Autodesk Fusion 360 part; units mm, degrees
note: some values were not read from the file. Set by a fixed rule: which sketch regions a step uses.
(part 13 of 15)
  line L10593 (41.7362, -55.8779) -> (41.8637, -56.1141)
  line L10594 (295.811, -57.5311) -> (295.669, -57.7588)
  line L10595 (295.496, -57.9642) -> (295.297, -58.1433)
  line L10596 (38.2329, -56.8363) -> (38.2603, -56.5693)
  line L10597 (42.0283, -57.0153) -> (41.9925, -57.2813)
  line L10598 (120.911, -58.0691) -> (121.001, -57.9066)
  line L10599 (41.3885, -55.4708) -> (41.5768, -55.662)
  line L10600 (292.292, -57.1145) -> (292.243, -56.8505)
  line L10601 (293.517, -58.4396) -> (293.269, -58.3349)
  line L10602 (-14.6725, -54.4815) -> (-14.3973, -54.5453)
  line L10603 (293.139, -55.022) -> (293.377, -54.8983)
  line L10604 (292.233, -56.5823) -> (292.26, -56.3153)
  line L10605 (-13.8873, -54.7853) -> (-13.6627, -54.9567)
  line L10606 (292.561, -55.574) -> (292.727, -55.3633)
  line L10607 (292.921, -55.178) -> (293.139, -55.022)
  line L10608 (292.377, -57.3691) -> (292.292, -57.1145)
  line L10609 (293.269, -58.3349) -> (293.039, -58.1965)
  line L10610 (295.297, -58.1433) -> (295.073, -58.2924)
  line L10611 (294.042, -58.5399) -> (293.776, -58.5083)
  line L10612 (294.311, -58.5336) -> (294.042, -58.5399)
  line L10613 (-14.3973, -54.5453) -> (-14.1338, -54.6473)
  line L10614 (292.727, -55.3633) -> (292.921, -55.178)
  line L10615 (292.497, -57.6092) -> (292.377, -57.3691)
  line L10616 (293.631, -54.8093) -> (293.894, -54.757)
  line L10617 (294.162, -54.7422) -> (294.429, -54.7654)
  line L10618 (-13.1625, -55.6339) -> (-13.0648, -55.8989)
  line L10619 (-13.0648, -55.8989) -> (-13.0053, -56.1751)
  line L10620 (-13.9944, -58.1942) -> (-14.2491, -58.3165)
  line L10621 (-16.5462, -57.7074) -> (-16.7068, -57.475)
  line L10622 (-16.7068, -57.475) -> (-16.8331, -57.2223)
  line L10623 (292.325, -56.0549) -> (292.426, -55.8061)
  line L10624 (292.26, -56.3153) -> (292.325, -56.0549)
  line L10625 (293.894, -54.757) -> (294.162, -54.7422)
  line L10626 (-13.1036, -57.1344) -> (-13.2178, -57.3928)
  line L10627 (-16.9225, -56.9543) -> (-16.9733, -56.6764)
  line L10628 (-13.5491, -57.8487) -> (-13.7595, -58.0372)
  line L10629 (293.776, -58.5083) -> (293.517, -58.4396)
  line L10630 (-14.2491, -58.3165) -> (-14.5185, -58.4016)
  line L10631 (294.576, -58.4895) -> (294.311, -58.5336)
  line L10632 (-16.8331, -57.2223) -> (-16.9225, -56.9543)
  line L10633 (-16.9733, -56.6764) -> (-16.9844, -56.3941)
  line L10634 (-16.9844, -56.3941) -> (-16.9556, -56.1131)
  line L10635 (-16.9556, -56.1131) -> (-16.8875, -55.8389)
  line L10636 (293.377, -54.8983) -> (293.631, -54.8093)
  line L10637 (39.6306, -55.0633) -> (39.8939, -55.011)
  line L10638 (295.577, -55.408) -> (295.736, -55.6239)
  line L10639 (293.039, -58.1965) -> (292.831, -58.027)
  line L10640 (295.073, -58.2924) -> (294.831, -58.4086)
  line L10641 (-13.0053, -56.1751) -> (-12.9853, -56.4569)
  line L10642 (292.831, -58.027) -> (292.649, -57.83)
  line L10643 (294.831, -58.4086) -> (294.576, -58.4895)
  line L10644 (-13.4645, -55.158) -> (-13.2967, -55.3853)
  line L10645 (-14.1338, -54.6473) -> (-13.8873, -54.7853)
  line L10646 (-16.8875, -55.8389) -> (-16.7814, -55.577)
  line L10647 (295.175, -55.054) -> (295.388, -55.2168)
  line L10648 (292.243, -56.8505) -> (292.233, -56.5823)
  line L10649 (292.649, -57.83) -> (292.497, -57.6092)
  line L10650 (292.426, -55.8061) -> (292.561, -55.574)
  line L10651 (38.2435, -57.1045) -> (38.2329, -56.8363)
  line L10652 (-9.0561, -57.5495) -> (-9.1147, -57.7254)
  line L10653 (-15.7796, -54.6214) -> (-15.5131, -54.5278)
  line L10654 (-9.0329, -57.3656) -> (-9.0561, -57.5495)
  line L10655 (-15.8933, -58.2389) -> (-16.1354, -58.0932)
  line L10656 (-13.7595, -58.0372) -> (-13.9944, -58.1942)
  line L10657 (-13.6627, -54.9567) -> (-13.4645, -55.158)
  line L10658 (-13.3673, -57.6325) -> (-13.5491, -57.8487)
  line L10659 (-10.5247, -58.1191) -> (-10.6659, -57.999)
  line L10660 (-16.6395, -55.3327) -> (-16.4646, -55.1109)
  line L10661 (-9.4735, -58.1412) -> (-9.639, -58.2248)
  line L10662 (-10.7811, -57.8537) -> (-10.8658, -57.6888)
  line L10663 (-9.1913, -56.8133) -> (-9.1042, -56.977)
  line L10664 (160.061, -56.6385) -> (160.163, -56.7784)
  line L10665 (-9.9759, -56.3891) -> (-9.7915, -56.4084)
  line L10666 (-9.0506, -57.1545) -> (-9.0325, -57.339)
  line L10667 (160.25, -57.2828) -> (160.2, -57.4491)
  line L10668 (160.2, -57.4491) -> (160.113, -57.5993)
  line L10669 (-9.4513, -56.5515) -> (-9.3084, -56.6696)
  line L10670 (-9.1147, -57.7254) -> (-9.2062, -57.8867)
  line L10671 (-9.639, -58.2248) -> (-9.8176, -58.2746)
  line L10672 (-10.3629, -58.2096) -> (-10.5247, -58.1191)
  line L10673 (158.251, -57.853) -> (158.096, -57.774)
  line L10674 (159.605, -56.4058) -> (159.773, -56.447)
  line L10675 (-10.9324, -57.3258) -> (-10.9118, -57.1415)
  line L10676 (-9.2062, -57.8867) -> (-9.3274, -58.027)
  line L10677 (158.419, -57.8942) -> (158.251, -57.853)
  line L10678 (158.096, -57.774) -> (157.963, -57.6615)
  line L10679 (160.163, -56.7784) -> (160.231, -56.9382)
  line L10680 (-16.2602, -54.9159) -> (-16.0303, -54.7516)
  line L10681 (-10.9118, -57.1415) -> (-10.8557, -56.9648)
  line L10682 (-13.2178, -57.3928) -> (-13.3673, -57.6325)
  line L10683 (-14.9539, -54.4572) -> (-14.6725, -54.4815)
  line L10684 (-9.1042, -56.977) -> (-9.0506, -57.1545)
  line L10685 (-15.5131, -54.5278) -> (-15.236, -54.4727)
  line L10686 (160.261, -57.1094) -> (160.25, -57.2828)
  line L10687 (157.963, -57.6615) -> (157.861, -57.5216)
  line L10688 (-9.6144, -56.4633) -> (-9.4513, -56.5515)
  line L10689 (160.231, -56.9382) -> (160.261, -57.1094)
  line L10690 (-16.0303, -54.7516) -> (-15.7796, -54.6214)
  line L10691 (-14.7971, -58.448) -> (-15.0796, -58.4547)
  line L10692 (-13.2967, -55.3853) -> (-13.1625, -55.6339)
  line L10693 (-15.6332, -58.3491) -> (-15.8933, -58.2389)
  line L10694 (-16.3544, -57.9148) -> (-16.5462, -57.7074)
  line L10695 (-12.9893, -56.5825) -> (-13.0269, -56.8625)
  line L10696 (-10.0024, -58.2888) -> (-10.1865, -58.2669)
  line L10697 (-14.5185, -58.4016) -> (-14.7971, -58.448)
  line L10698 (-12.9853, -56.4569) -> (-12.9893, -56.5825)
  line L10699 (-16.7814, -55.577) -> (-16.6395, -55.3327)
  line L10700 (-10.1865, -58.2669) -> (-10.3629, -58.2096)
  line L10701 (-9.3084, -56.6696) -> (-9.1913, -56.8133)
  line L10702 (-10.8658, -57.6888) -> (-10.9169, -57.5105)
  line L10703 (-9.0325, -57.339) -> (-9.0329, -57.3656)
  line L10704 (-15.236, -54.4727) -> (-14.9539, -54.4572)
  line L10705 (-9.3274, -58.027) -> (-9.4735, -58.1412)
  line L10706 (-10.6659, -57.999) -> (-10.7811, -57.8537)
  line L10707 (-10.7664, -56.8023) -> (-10.6472, -56.6603)
  line L10708 (-9.8176, -58.2746) -> (-10.0024, -58.2888)
  line L10709 (-10.3384, -56.4582) -> (-10.1605, -56.4059)
  line L10710 (-15.0796, -58.4547) -> (-15.3601, -58.4215)
  line L10711 (-16.1354, -58.0932) -> (-16.3544, -57.9148)
  line L10712 (-9.7915, -56.4084) -> (-9.6144, -56.4633)
  line L10713 (-16.4646, -55.1109) -> (-16.2602, -54.9159)
  line L10714 (-13.0269, -56.8625) -> (-13.1036, -57.1344)
  line L10715 (-15.3601, -58.4215) -> (-15.6332, -58.3491)
  line L10716 (174.033, -57.3618) -> (174.003, -57.1906)
  line L10717 (-20.7867, -56.0894) -> (-20.8715, -55.9245)
  line L10718 (157.911, -56.7007) -> (158.031, -56.5746)
  line L10719 (-19.6446, -56.4605) -> (-19.8232, -56.5103)
  line L10720 (176.168, -56.526) -> (176.301, -56.6385)
  line L10721 (-19.1099, -55.2128) -> (-19.0563, -55.3903)
  line L10722 (176.013, -56.447) -> (176.168, -56.526)
  line L10723 (174.752, -56.4) -> (175.752, -56.4)
  line L10724 (-20.0081, -56.5246) -> (-20.1922, -56.5026)
  line L10725 (157.793, -57.3618) -> (157.763, -57.1906)
  line L10726 (-19.62, -54.699) -> (-19.4569, -54.7872)
  line L10727 (174.014, -57.0172) -> (174.064, -56.8509)
  line L10728 (-20.6715, -56.2347) -> (-20.7867, -56.0894)
  line L10729 (-20.8715, -55.9245) -> (-20.9226, -55.7463)
  line L10730 (176.088, -57.8206) -> (175.925, -57.8799)
  line L10731 (-19.1969, -55.0491) -> (-19.1099, -55.2128)
  line L10732 (157.763, -57.1906) -> (157.774, -57.0172)
  line L10733 (160.113, -57.5993) -> (159.993, -57.7254)
  line L10734 (176.403, -56.7784) -> (176.471, -56.9382)
  line L10735 (176.301, -56.6385) -> (176.403, -56.7784)
  line L10736 (159.993, -57.7254) -> (159.848, -57.8206)
  line L10737 (-10.1605, -56.4059) -> (-9.9759, -56.3891)
  line L10738 (159.512, -56.4) -> (159.605, -56.4058)
  line L10739 (174.064, -56.8509) -> (174.151, -56.7007)
  line L10740 (174.003, -57.1906) -> (174.014, -57.0172)
  line L10741 (159.848, -57.8206) -> (159.685, -57.8799)
  line L10742 (175.925, -57.8799) -> (175.752, -57.9)
  line L10743 (174.752, -57.9) -> (174.659, -57.8942)
  line L10744 (159.773, -56.447) -> (159.928, -56.526)
  line L10745 (174.336, -57.774) -> (174.203, -57.6615)
  line L10746 (158.512, -56.4) -> (159.512, -56.4)
  line L10747 (174.491, -57.853) -> (174.336, -57.774)
  line L10748 (158.339, -56.4201) -> (158.512, -56.4)
  line L10749 (176.471, -56.9382) -> (176.501, -57.1094)
  line L10750 (175.752, -57.9) -> (174.752, -57.9)
  line L10751 (-19.3141, -54.9054) -> (-19.1969, -55.0491)
  line L10752 (158.031, -56.5746) -> (158.176, -56.4794)
  line L10753 (-10.8557, -56.9648) -> (-10.7664, -56.8023)
  line L10754 (176.233, -57.7254) -> (176.088, -57.8206)
  line L10755 (-19.0563, -55.3903) -> (-19.0382, -55.5748)
  line L10756 (157.824, -56.8509) -> (157.911, -56.7007)
  line L10757 (174.416, -56.4794) -> (174.579, -56.4201)
  line L10758 (175.845, -56.4058) -> (176.013, -56.447)
  line L10759 (174.659, -57.8942) -> (174.491, -57.853)
  line L10760 (174.579, -56.4201) -> (174.752, -56.4)
  line L10761 (159.685, -57.8799) -> (159.512, -57.9)
  line L10762 (-10.5027, -56.5441) -> (-10.3384, -56.4582)
  line L10763 (-10.9169, -57.5105) -> (-10.9324, -57.3258)
  line L10764 (158.512, -57.9) -> (158.419, -57.8942)
  line L10765 (174.203, -57.6615) -> (174.101, -57.5216)
  line L10766 (176.49, -57.2828) -> (176.44, -57.4491)
  line L10767 (176.501, -57.1094) -> (176.49, -57.2828)
  line L10768 (176.44, -57.4491) -> (176.353, -57.5993)
  line L10769 (159.928, -56.526) -> (160.061, -56.6385)
  line L10770 (158.176, -56.4794) -> (158.339, -56.4201)
  line L10771 (174.101, -57.5216) -> (174.033, -57.3618)
  line L10772 (174.271, -56.5746) -> (174.416, -56.4794)
  line L10773 (-19.4791, -56.3769) -> (-19.6446, -56.4605)
  line L10774 (157.861, -57.5216) -> (157.793, -57.3618)
  line L10775 (-19.1203, -55.9612) -> (-19.2119, -56.1224)
  line L10776 (157.774, -57.0172) -> (157.824, -56.8509)
  line L10777 (159.512, -57.9) -> (158.512, -57.9)
  line L10778 (176.353, -57.5993) -> (176.233, -57.7254)
  line L10779 (-10.6472, -56.6603) -> (-10.5027, -56.5441)
  line L10780 (227.851, -53.2483) -> (227.911, -53.5245)
  line L10781 (226.667, -55.6658) -> (226.398, -55.751)
  line L10782 (-20.5084, -54.7799) -> (-20.344, -54.694)
  line L10783 (224.562, -55.2642) -> (224.37, -55.0568)
  line L10784 (174.151, -56.7007) -> (174.271, -56.5746)
  line L10785 (-20.9174, -55.3773) -> (-20.8614, -55.2005)
  line L10786 (227.931, -53.8063) -> (227.927, -53.9318)
  line L10787 (-20.5304, -56.3549) -> (-20.6715, -56.2347)
  line L10788 (225.023, -55.5883) -> (224.781, -55.4426)
  line L10789 (-19.0382, -55.5748) -> (-19.0385, -55.6013)
  line L10790 (225.283, -55.6984) -> (225.023, -55.5883)
  line L10791 (110.112, -52.6945) -> (110.247, -52.9432)
  line L10792 (110.344, -53.2082) -> (110.404, -53.4844)
  line L10793 (223.961, -53.4624) -> (224.029, -53.1882)
  line L10794 (109.746, -52.266) -> (109.945, -52.4673)
  line L10795 (110.404, -53.4844) -> (110.424, -53.7662)
  line L10796 (226.119, -55.7974) -> (225.837, -55.804)
  line L10797 (227.029, -52.1347) -> (227.253, -52.306)
  line L10798 (224.451, -52.4602) -> (224.656, -52.2652)
  line L10799 (224.781, -55.4426) -> (224.562, -55.2642)
  line L10800 (227.253, -52.306) -> (227.452, -52.5074)
  line L10801 (227.452, -52.5074) -> (227.619, -52.7346)
  line L10802 (226.782, -51.9966) -> (227.029, -52.1347)
  line L10803 (-20.6529, -54.896) -> (-20.5084, -54.7799)
  line L10804 (224.277, -52.6821) -> (224.451, -52.4602)
  line L10805 (225.837, -55.804) -> (225.556, -55.7708)
  line L10806 (-20.1662, -54.6416) -> (-19.9815, -54.6248)
  line L10807 (109.945, -52.4673) -> (110.112, -52.6945)
  line L10808 (-19.0618, -55.7852) -> (-19.1203, -55.9612)
  line L10809 (-20.9226, -55.7463) -> (-20.9381, -55.5615)
  line L10810 (-20.8614, -55.2005) -> (-20.772, -55.0381)
  line L10811 (227.549, -54.9818) -> (227.367, -55.1981)
  line L10812 (223.994, -54.3036) -> (223.943, -54.0257)
  line L10813 (225.68, -51.822) -> (225.962, -51.8065)
  line L10814 (227.889, -54.2118) -> (227.812, -54.4837)
  line L10815 (225.962, -51.8065) -> (226.244, -51.8309)
  line L10816 (226.398, -55.751) -> (226.119, -55.7974)
  line L10817 (227.911, -53.5245) -> (227.931, -53.8063)
  line L10818 (-19.0385, -55.6013) -> (-19.0618, -55.7852)
  line L10819 (-19.333, -56.2627) -> (-19.4791, -56.3769)
  line L10820 (-19.7971, -54.6442) -> (-19.62, -54.699)
  line L10821 (226.922, -55.5435) -> (226.667, -55.6658)
  line L10822 (225.556, -55.7708) -> (225.283, -55.6984)
  line L10823 (-20.772, -55.0381) -> (-20.6529, -54.896)
  line L10824 (227.157, -55.3866) -> (226.922, -55.5435)
  line L10825 (-19.8232, -56.5103) -> (-20.0081, -56.5246)
  line L10826 (-20.1922, -56.5026) -> (-20.3685, -56.4453)
  line L10827 (227.367, -55.1981) -> (227.157, -55.3866)
  line L10828 (226.519, -51.8947) -> (226.782, -51.9966)
  line L10829 (109.275, -51.9565) -> (109.522, -52.0946)
  line L10830 (-19.9815, -54.6248) -> (-19.7971, -54.6442)
  line L10831 (-20.344, -54.694) -> (-20.1662, -54.6416)
  line L10832 (227.812, -54.4837) -> (227.698, -54.7421)
  line L10833 (175.752, -56.4) -> (175.845, -56.4058)
  line L10834 (227.754, -52.9832) -> (227.851, -53.2483)
  line L10835 (226.244, -51.8309) -> (226.519, -51.8947)
  line L10836 (227.698, -54.7421) -> (227.549, -54.9818)
  line L10837 (110.247, -52.9432) -> (110.344, -53.2082)
  line L10838 (-19.2119, -56.1224) -> (-19.333, -56.2627)
  line L10839 (-19.4569, -54.7872) -> (-19.3141, -54.9054)
  line L10840 (227.619, -52.7346) -> (227.754, -52.9832)
  line L10841 (227.927, -53.9318) -> (227.889, -54.2118)
  line L10842 (-20.9381, -55.5615) -> (-20.9174, -55.3773)
  line L10843 (-20.3685, -56.4453) -> (-20.5304, -56.3549)
  line L10844 (106.487, -54.2636) -> (106.436, -53.9857)
  line L10845 (108.612, -55.7573) -> (108.33, -55.764)
  line L10846 (224.135, -52.9264) -> (224.277, -52.6821)
  line L10847 (223.932, -53.7434) -> (223.961, -53.4624)
  line L10848 (224.886, -52.101) -> (225.136, -51.9708)
  line L10849 (106.576, -54.5316) -> (106.487, -54.2636)
  line L10850 (107.516, -55.5482) -> (107.274, -55.4025)
  line L10851 (108.891, -55.7109) -> (108.612, -55.7573)
  line L10852 (108.455, -51.7664) -> (108.737, -51.7908)
  line L10853 (108.173, -51.782) -> (108.455, -51.7664)
  line L10854 (221.806, -54.3264) -> (221.86, -54.5039)
  line L10855 (110.42, -53.8918) -> (110.382, -54.1718)
  line L10856 (221.86, -54.5039) -> (221.878, -54.6884)
  line L10857 (221.296, -53.8126) -> (221.459, -53.9008)
  line L10858 (219.978, -54.6751) -> (219.999, -54.4909)
  line L10859 (220.144, -54.1517) -> (220.263, -54.0097)
  line L10860 (108.33, -55.764) -> (108.049, -55.7308)
  line L10861 (225.136, -51.9708) -> (225.403, -51.8772)
  line L10862 (106.522, -53.1482) -> (106.628, -52.8863)
  line L10863 (221.459, -53.9008) -> (221.602, -54.019)
  line L10864 (110.382, -54.1718) -> (110.306, -54.4437)
  line L10865 (106.436, -53.9857) -> (106.425, -53.7034)
  line L10866 (221.878, -54.6884) -> (221.878, -54.7149)
  line L10867 (110.042, -54.9418) -> (109.86, -55.158)
  line L10868 (221.437, -55.4905) -> (221.271, -55.5741)
  line L10869 (223.943, -54.0257) -> (223.932, -53.7434)
  line L10870 (107.055, -55.2241) -> (106.863, -55.0167)
  line L10871 (221.093, -55.624) -> (220.908, -55.6382)
  line L10872 (110.424, -53.7662) -> (110.42, -53.8918)
  line L10873 (110.306, -54.4437) -> (110.191, -54.7021)
  line L10874 (106.454, -53.4223) -> (106.522, -53.1482)
  line L10875 (106.77, -52.642) -> (106.945, -52.4202)
  line L10876 (220.263, -54.0097) -> (220.408, -53.8935)
  line L10877 (220.045, -55.0381) -> (219.994, -54.8599)
  line L10878 (220.408, -53.8935) -> (220.572, -53.8076)
  line L10879 (220.055, -54.3142) -> (220.144, -54.1517)
  line L10880 (110.191, -54.7021) -> (110.042, -54.9418)
  line L10881 (106.945, -52.4202) -> (107.149, -52.2252)
  line L10882 (224.029, -53.1882) -> (224.135, -52.9264)
  line L10883 (106.425, -53.7034) -> (106.454, -53.4223)
  line L10884 (107.776, -55.6584) -> (107.516, -55.5482)
  line L10885 (108.737, -51.7908) -> (109.012, -51.8546)
  line L10886 (106.628, -52.8863) -> (106.77, -52.642)
  line L10887 (106.702, -54.7843) -> (106.576, -54.5316)
  line L10888 (107.896, -51.8371) -> (108.173, -51.782)
  line L10889 (109.522, -52.0946) -> (109.746, -52.266)
  line L10890 (107.629, -51.9307) -> (107.896, -51.8371)
  line L10891 (225.403, -51.8772) -> (225.68, -51.822)
  line L10892 (109.012, -51.8546) -> (109.275, -51.9565)
  line L10893 (224.083, -54.5716) -> (223.994, -54.3036)
  line L10894 (109.86, -55.158) -> (109.65, -55.3465)
  line L10895 (109.65, -55.3465) -> (109.415, -55.5035)
  line L10896 (108.049, -55.7308) -> (107.776, -55.6584)
  line L10897 (109.415, -55.5035) -> (109.16, -55.6258)
  line L10898 (107.379, -52.0609) -> (107.629, -51.9307)
  line L10899 (221.271, -55.5741) -> (221.093, -55.624)
  line L10900 (224.656, -52.2652) -> (224.886, -52.101)
  line L10901 (219.999, -54.4909) -> (220.055, -54.3142)
  line L10902 (107.149, -52.2252) -> (107.379, -52.0609)
  line L10903 (224.37, -55.0568) -> (224.209, -54.8243)
  line L10904 (106.863, -55.0167) -> (106.702, -54.7843)
  line L10905 (107.274, -55.4025) -> (107.055, -55.2241)
  line L10906 (224.209, -54.8243) -> (224.083, -54.5716)
  line L10907 (109.16, -55.6258) -> (108.891, -55.7109)
  line L10908 (114.203, -55.1959) -> (114.082, -55.3363)
  line L10909 (159.605, -53.8658) -> (159.773, -53.907)
  line L10910 (112.643, -54.1116) -> (112.762, -53.9696)
  line L10911 (221.719, -54.1627) -> (221.806, -54.3264)
  line L10912 (220.724, -55.6162) -> (220.548, -55.5589)
  line L10913 (221.878, -54.7149) -> (221.854, -54.8989)
  line L10914 (220.935, -53.7384) -> (221.119, -53.7578)
  line L10915 (112.497, -54.4508) -> (112.553, -54.2741)
  line L10916 (220.75, -53.7552) -> (220.935, -53.7384)
  line L10917 (112.477, -54.6351) -> (112.497, -54.4508)
  line L10918 (157.861, -54.9816) -> (157.793, -54.8218)
  line L10919 (112.553, -54.2741) -> (112.643, -54.1116)
  line L10920 (160.061, -54.0985) -> (160.163, -54.2384)
  line L10921 (113.071, -53.7675) -> (113.249, -53.7152)
  line L10922 (112.743, -55.3083) -> (112.628, -55.163)
  line L10923 (159.512, -55.36) -> (158.512, -55.36)
  line L10924 (157.793, -54.8218) -> (157.763, -54.6506)
  line L10925 (219.994, -54.8599) -> (219.978, -54.6751)
  line L10926 (113.046, -55.5189) -> (112.884, -55.4284)
  line L10927 (113.618, -53.7177) -> (113.795, -53.7726)
  line L10928 (112.906, -53.8534) -> (113.071, -53.7675)
  line L10929 (157.763, -54.6506) -> (157.774, -54.4772)
  line L10930 (159.993, -55.1854) -> (159.848, -55.2806)
  line L10931 (113.407, -55.5981) -> (113.223, -55.5762)
  line L10932 (113.936, -55.4504) -> (113.77, -55.534)
  line L10933 (220.386, -55.4685) -> (220.245, -55.3483)
  line L10934 (113.592, -55.5839) -> (113.407, -55.5981)
  line L10935 (157.824, -54.3109) -> (157.911, -54.1607)
  line L10936 (114.305, -54.2863) -> (114.359, -54.4638)
  line L10937 (157.963, -55.1215) -> (157.861, -54.9816)
  line L10938 (221.119, -53.7578) -> (221.296, -53.8126)
  line L10939 (114.377, -54.6483) -> (114.376, -54.6749)
  line L10940 (114.218, -54.1226) -> (114.305, -54.2863)
  line L10941 (113.958, -53.8607) -> (114.101, -53.9789)
  line L10942 (220.548, -55.5589) -> (220.386, -55.4685)
  line L10943 (157.774, -54.4772) -> (157.824, -54.3109)
  line L10944 (220.908, -55.6382) -> (220.724, -55.6162)
  line L10945 (159.773, -53.907) -> (159.928, -53.986)
  line L10946 (113.77, -55.534) -> (113.592, -55.5839)
  line L10947 (221.854, -54.8989) -> (221.796, -55.0748)
  line L10948 (221.583, -55.3764) -> (221.437, -55.4905)
  line L10949 (220.572, -53.8076) -> (220.75, -53.7552)
  line L10950 (221.704, -55.236) -> (221.583, -55.3764)
  line L10951 (112.884, -55.4284) -> (112.743, -55.3083)
  line L10952 (114.353, -54.8588) -> (114.294, -55.0347)
  line L10953 (221.796, -55.0748) -> (221.704, -55.236)
  line L10954 (114.101, -53.9789) -> (114.218, -54.1226)
  line L10955 (113.223, -55.5762) -> (113.046, -55.5189)
  line L10956 (112.492, -54.8198) -> (112.477, -54.6351)
  line L10957 (114.376, -54.6749) -> (114.353, -54.8588)
  line L10958 (114.294, -55.0347) -> (114.203, -55.1959)
  line L10959 (113.795, -53.7726) -> (113.958, -53.8607)
  line L10960 (158.096, -55.234) -> (157.963, -55.1215)
  line L10961 (160.113, -55.0593) -> (159.993, -55.1854)
  line L10962 (114.359, -54.4638) -> (114.377, -54.6483)
  line L10963 (159.848, -55.2806) -> (159.685, -55.3399)
  line L10964 (112.628, -55.163) -> (112.543, -54.9981)
  line L10965 (159.928, -53.986) -> (160.061, -54.0985)
  line L10966 (220.245, -55.3483) -> (220.129, -55.203)
  line L10967 (220.129, -55.203) -> (220.045, -55.0381)
  line L10968 (112.543, -54.9981) -> (112.492, -54.8198)
  line L10969 (114.082, -55.3363) -> (113.936, -55.4504)
  line L10970 (221.602, -54.019) -> (221.719, -54.1627)
  line L10971 (112.762, -53.9696) -> (112.906, -53.8534)
  line L10972 (176.501, -54.5694) -> (176.49, -54.7428)
  line L10973 (-32.6479, -51.4773) -> (-32.4233, -51.6487)
  line L10974 (-33.0097, -55.0085) -> (-33.279, -55.0937)
  line L10975 (-34.1207, -55.1135) -> (-34.3938, -55.0411)
  line L10976 (-31.8254, -52.5909) -> (-31.7659, -52.8671)
  line L10977 (176.49, -54.7428) -> (176.44, -54.9091)
  line L10978 (-32.2251, -51.85) -> (-32.0573, -52.0773)
  line L10979 (-34.3938, -55.0411) -> (-34.6539, -54.9309)
  line L10980 (-31.7459, -53.1489) -> (-31.7499, -53.2745)
  line L10981 (158.031, -54.0346) -> (158.176, -53.9394)
  line L10982 (176.301, -54.0985) -> (176.403, -54.2384)
  line L10983 (-34.6539, -54.9309) -> (-34.8959, -54.7852)
  line L10984 (-31.7875, -53.5545) -> (-31.8642, -53.8264)
  line L10985 (174.659, -55.3542) -> (174.491, -55.313)
  line L10986 (175.752, -55.36) -> (174.752, -55.36)
  line L10987 (-34.8959, -54.7852) -> (-35.115, -54.6068)
  line L10988 (160.25, -54.7428) -> (160.2, -54.9091)
  line L10989 (160.231, -54.3982) -> (160.261, -54.5694)
  line L10990 (175.752, -53.86) -> (175.845, -53.8658)
  line L10991 (174.752, -53.86) -> (175.752, -53.86)
  line L10992 (160.261, -54.5694) -> (160.25, -54.7428)
  line L10993 (158.251, -55.313) -> (158.096, -55.234)
  line L10994 (175.845, -53.8658) -> (176.013, -53.907)
  line L10995 (174.752, -55.36) -> (174.659, -55.3542)
  line L10996 (176.471, -54.3982) -> (176.501, -54.5694)
  line L10997 (158.512, -53.86) -> (159.512, -53.86)
  line L10998 (176.168, -53.986) -> (176.301, -54.0985)
  line L10999 (-32.755, -54.8862) -> (-33.0097, -55.0085)
  line L11000 (113.433, -53.6984) -> (113.618, -53.7177)
  line L11001 (176.013, -53.907) -> (176.168, -53.986)
  line L11002 (-32.4233, -51.6487) -> (-32.2251, -51.85)
  line L11003 (174.101, -54.9816) -> (174.033, -54.8218)
  line L11004 (-33.4331, -51.1735) -> (-33.1579, -51.2373)
  line L11005 (-31.8642, -53.8264) -> (-31.9784, -54.0848)
  line L11006 (174.064, -54.3109) -> (174.151, -54.1607)
  line L11007 (174.336, -55.234) -> (174.203, -55.1215)
  line L11008 (174.151, -54.1607) -> (174.271, -54.0346)
  line L11009 (113.249, -53.7152) -> (113.433, -53.6984)
  line L11010 (174.491, -55.313) -> (174.336, -55.234)
  line L11011 (174.014, -54.4772) -> (174.064, -54.3109)
  line L11012 (160.2, -54.9091) -> (160.113, -55.0593)
  line L11013 (174.271, -54.0346) -> (174.416, -53.9394)
  line L11014 (174.003, -54.6506) -> (174.014, -54.4772)
  line L11015 (176.44, -54.9091) -> (176.353, -55.0593)
  line L11016 (176.088, -55.2806) -> (175.925, -55.3399)
  line L11017 (157.911, -54.1607) -> (158.031, -54.0346)
  line L11018 (158.419, -55.3542) -> (158.251, -55.313)
  line L11019 (160.163, -54.2384) -> (160.231, -54.3982)
  line L11020 (174.033, -54.8218) -> (174.003, -54.6506)
  line L11021 (174.579, -53.8801) -> (174.752, -53.86)
  line L11022 (176.233, -55.1854) -> (176.088, -55.2806)
  line L11023 (158.512, -55.36) -> (158.419, -55.3542)
  line L11024 (176.353, -55.0593) -> (176.233, -55.1854)
  line L11025 (158.339, -53.8801) -> (158.512, -53.86)
  line L11026 (175.925, -55.3399) -> (175.752, -55.36)
  line L11027 (176.403, -54.2384) -> (176.471, -54.3982)
  line L11028 (174.203, -55.1215) -> (174.101, -54.9816)
  line L11029 (-31.9231, -52.3259) -> (-31.8254, -52.5909)
  line L11030 (-35.3068, -54.3994) -> (-35.4674, -54.167)
  line L11031 (-31.7499, -53.2745) -> (-31.7875, -53.5545)
  line L11032 (174.416, -53.9394) -> (174.579, -53.8801)
  line L11033 (159.685, -55.3399) -> (159.512, -55.36)
  line L11034 (159.512, -53.86) -> (159.605, -53.8658)
  line L11035 (158.176, -53.9394) -> (158.339, -53.8801)
  line L11036 (-35.4001, -52.0247) -> (-35.2252, -51.8029)
  line L11037 (-33.7145, -51.1492) -> (-33.4331, -51.1735)
  line L11038 (-33.279, -55.0937) -> (-33.5577, -55.14)
  line L11039 (-35.6481, -52.5309) -> (-35.542, -52.269)
  line L11040 (-28.2341, -54.8332) -> (-28.3996, -54.9168)
  line L11041 (-27.8752, -54.4174) -> (-27.9668, -54.5787)
  line L11042 (-27.9668, -54.5787) -> (-28.088, -54.719)
  line L11043 (-35.2252, -51.8029) -> (-35.0208, -51.6079)
  line L11044 (-28.7365, -53.0811) -> (-28.5521, -53.1004)
  line L11045 (231.865, -52.7396) -> (231.884, -52.9241)
  line L11046 (-28.5521, -53.1004) -> (-28.375, -53.1553)
  line L11047 (231.801, -53.3105) -> (231.71, -53.4717)
  line L11048 (230.914, -53.8739) -> (230.73, -53.852)
  line L11049 (-29.527, -53.4943) -> (-29.4078, -53.3523)
  line L11050 (-29.2853, -54.8111) -> (-29.4265, -54.691)
  line L11051 (231.589, -53.6121) -> (231.443, -53.7262)
  line L11052 (-28.9211, -53.0979) -> (-28.7365, -53.0811)
  line L11053 (-28.9471, -54.9589) -> (-29.1234, -54.9016)
  line L11054 (-32.1279, -54.3245) -> (-32.3097, -54.5407)
  line L11055 (-35.542, -52.269) -> (-35.4001, -52.0247)
  line L11056 (-27.8167, -54.2415) -> (-27.8752, -54.4174)
  line L11057 (-29.2633, -53.2361) -> (-29.099, -53.1502)
  line L11058 (231.099, -53.8597) -> (230.914, -53.8739)
  line L11059 (-29.693, -54.0178) -> (-29.6724, -53.8335)
  line L11060 (-35.115, -54.6068) -> (-35.3068, -54.3994)
  line L11061 (-28.375, -53.1553) -> (-28.2119, -53.2435)
  line L11062 (-33.1579, -51.2373) -> (-32.8944, -51.3393)
  line L11063 (-29.4078, -53.3523) -> (-29.2633, -53.2361)
  line L11064 (-27.9518, -53.5053) -> (-27.8648, -53.669)
  line L11065 (-33.5577, -55.14) -> (-33.8402, -55.1467)
  line L11066 (-35.6831, -53.6463) -> (-35.7339, -53.3684)
  line L11067 (-35.7339, -53.3684) -> (-35.745, -53.0861)
  line L11068 (-34.7909, -51.4436) -> (-34.5402, -51.3134)
  line L11069 (-35.7162, -52.8051) -> (-35.6481, -52.5309)
  line L11070 (-35.5937, -53.9143) -> (-35.6831, -53.6463)
  line L11071 (-34.5402, -51.3134) -> (-34.2737, -51.2198)
  line L11072 (-33.9966, -51.1647) -> (-33.7145, -51.1492)
  line L11073 (-32.8944, -51.3393) -> (-32.6479, -51.4773)
  line L11074 (-33.8402, -55.1467) -> (-34.1207, -55.1135)
  line L11075 (-34.2737, -51.2198) -> (-33.9966, -51.1647)
  line L11076 (-28.2119, -53.2435) -> (-28.069, -53.3616)
  line L11077 (-29.5417, -54.5457) -> (-29.6264, -54.3808)
  line L11078 (-29.6724, -53.8335) -> (-29.6163, -53.6568)
  line L11079 (-29.6264, -54.3808) -> (-29.6775, -54.2025)
  line L11080 (231.884, -52.9241) -> (231.883, -52.9507)
  line L11081 (-35.4674, -54.167) -> (-35.5937, -53.9143)
  line L11082 (-27.7935, -54.0576) -> (-27.8167, -54.2415)
  line L11083 (230.73, -53.852) -> (230.553, -53.7947)
  line L11084 (-32.0573, -52.0773) -> (-31.9231, -52.3259)
  line L11085 (-28.088, -54.719) -> (-28.2341, -54.8332)
  line L11086 (-31.7659, -52.8671) -> (-31.7459, -53.1489)
  line L11087 (-32.3097, -54.5407) -> (-32.5201, -54.7292)
  line L11088 (-27.8112, -53.8465) -> (-27.7931, -54.031)
  line L11089 (-32.5201, -54.7292) -> (-32.755, -54.8862)
  line L11090 (-35.0208, -51.6079) -> (-34.7909, -51.4436)
  line L11091 (-31.9784, -54.0848) -> (-32.1279, -54.3245)
  line L11092 (-27.8648, -53.669) -> (-27.8112, -53.8465)
  line L11093 (-27.7931, -54.031) -> (-27.7935, -54.0576)
  line L11094 (-28.763, -54.9808) -> (-28.9471, -54.9589)
  line L11095 (-28.3996, -54.9168) -> (-28.5781, -54.9666)
  line L11096 (-28.069, -53.3616) -> (-27.9518, -53.5053)
  line L11097 (-29.1234, -54.9016) -> (-29.2853, -54.8111)
  line L11098 (-28.5781, -54.9666) -> (-28.763, -54.9808)
  line L11099 (-35.745, -53.0861) -> (-35.7162, -52.8051)
  line L11100 (103.952, -52.0965) -> (104.095, -52.2147)
  line L11101 (-29.099, -53.1502) -> (-28.9211, -53.0979)
  line L11102 (231.465, -52.1365) -> (231.608, -52.2547)
  line L11103 (104.076, -53.572) -> (103.93, -53.6862)
  line L11104 (104.289, -53.2705) -> (104.197, -53.4317)
  line L11105 (102.622, -53.3987) -> (102.538, -53.2338)
  line L11106 (102.538, -53.2338) -> (102.487, -53.0556)
  line L11107 (104.212, -52.3583) -> (104.299, -52.5221)
  line L11108 (-38.2397, -53.0689) -> (-38.4052, -53.1525)
  line L11109 (230.413, -52.1292) -> (230.578, -52.0433)
  line L11110 (-38.4052, -53.1525) -> (-38.5838, -53.2023)
  line L11111 (-38.5838, -53.2023) -> (-38.7687, -53.2166)
  line L11112 (-37.8809, -52.6532) -> (-37.9725, -52.8144)
  line L11113 (-38.7687, -53.2166) -> (-38.9528, -53.1946)
  line L11114 (230.756, -51.991) -> (230.94, -51.9742)
  line L11115 (102.901, -52.0891) -> (103.065, -52.0032)
  line L11116 (-37.8704, -51.9048) -> (-37.8169, -52.0823)
  line L11117 (104.347, -53.0945) -> (104.289, -53.2705)
  line L11118 (231.125, -51.9935) -> (231.302, -52.0484)
  line L11119 (104.197, -53.4317) -> (104.076, -53.572)
  line L11120 (103.586, -53.8196) -> (103.401, -53.8339)
  line L11121 (102.879, -53.6642) -> (102.738, -53.544)
  line L11122 (102.548, -52.5098) -> (102.637, -52.3473)
  line L11123 (102.637, -52.3473) -> (102.756, -52.2053)
  line L11124 (231.725, -52.3984) -> (231.812, -52.5621)
  line L11125 (104.371, -52.9106) -> (104.347, -53.0945)
  line L11126 (231.277, -53.8098) -> (231.099, -53.8597)
  line L11127 (-38.0747, -51.5974) -> (-37.9575, -51.7411)
  line L11128 (230.391, -53.7042) -> (230.25, -53.5841)
  line L11129 (-29.4265, -54.691) -> (-29.5417, -54.5457)
  line L11130 (229.999, -53.0956) -> (229.984, -52.9109)
  line L11131 (229.984, -52.9109) -> (230.004, -52.7266)
  line L11132 (231.71, -53.4717) -> (231.589, -53.6121)
  line L11133 (230.05, -53.2739) -> (229.999, -53.0956)
  line L11134 (231.883, -52.9507) -> (231.86, -53.1346)
  line L11135 (104.095, -52.2147) -> (104.212, -52.3583)
  line L11136 (230.15, -52.3874) -> (230.269, -52.2454)
  line L11137 (231.608, -52.2547) -> (231.725, -52.3984)
  line L11138 (231.86, -53.1346) -> (231.801, -53.3105)
  line L11139 (104.299, -52.5221) -> (104.353, -52.6995)
  line L11140 (230.25, -53.5841) -> (230.135, -53.4388)
  line L11141 (103.401, -53.8339) -> (103.217, -53.8119)
  line L11142 (103.217, -53.8119) -> (103.041, -53.7546)
  line L11143 (102.492, -52.6866) -> (102.548, -52.5098)
  line L11144 (-38.3806, -51.391) -> (-38.2175, -51.4792)
  line L11145 (230.553, -53.7947) -> (230.391, -53.7042)
  line L11146 (103.789, -52.0083) -> (103.952, -52.0965)
  line L11147 (-38.2175, -51.4792) -> (-38.0747, -51.5974)
  line L11148 (231.443, -53.7262) -> (231.277, -53.8098)
  line L11149 (230.578, -52.0433) -> (230.756, -51.991)
  line L11150 (-29.6775, -54.2025) -> (-29.693, -54.0178)
  line L11151 (231.812, -52.5621) -> (231.865, -52.7396)
  line L11152 (103.93, -53.6862) -> (103.765, -53.7698)
  line L11153 (-29.6163, -53.6568) -> (-29.527, -53.4943)
  line L11154 (230.135, -53.4388) -> (230.05, -53.2739)
  line L11155 (231.302, -52.0484) -> (231.465, -52.1365)
  line L11156 (230.269, -52.2454) -> (230.413, -52.1292)
  line L11157 (103.612, -51.9535) -> (103.789, -52.0083)
  line L11158 (104.353, -52.6995) -> (104.371, -52.8841)
  line L11159 (103.765, -53.7698) -> (103.586, -53.8196)
  line L11160 (230.94, -51.9742) -> (231.125, -51.9935)
  line L11161 (230.06, -52.5499) -> (230.15, -52.3874)
  line L11162 (104.371, -52.8841) -> (104.371, -52.9106)
  line L11163 (230.004, -52.7266) -> (230.06, -52.5499)
  line L11164 (-52.0396, -51.7857) -> (-52.3183, -51.832)
  line L11165 (-53.5515, -48.1356) -> (-53.3008, -48.0054)
  line L11166 (-51.1839, -48.3407) -> (-50.9857, -48.542)
  line L11167 (103.428, -51.9341) -> (103.612, -51.9535)
  line L11168 (-37.9575, -51.7411) -> (-37.8704, -51.9048)
  line L11169 (-37.7988, -52.2668) -> (-37.7991, -52.2933)
  line L11170 (102.471, -52.8708) -> (102.492, -52.6866)
  line L11171 (-50.6248, -50.5184) -> (-50.739, -50.7768)
  line L11172 (-39.5473, -52.7814) -> (-39.632, -52.6165)
  line L11173 (-38.7421, -51.3168) -> (-38.5577, -51.3362)
  line L11174 (-52.1937, -47.8655) -> (-51.9184, -47.9293)
  line L11175 (-39.2909, -53.0469) -> (-39.4321, -52.9267)
  line L11176 (-50.5105, -49.9665) -> (-50.5481, -50.2465)
  line L11177 (-53.9858, -48.4949) -> (-53.7814, -48.2999)
  line L11178 (-51.655, -48.0313) -> (-51.4085, -48.1693)
  line L11179 (-54.228, -50.859) -> (-54.3543, -50.6063)
  line L11180 (-53.3008, -48.0054) -> (-53.0343, -47.9118)
  line L11181 (-39.632, -52.6165) -> (-39.6832, -52.4383)
  line L11182 (-50.8179, -48.7693) -> (-50.6837, -49.0179)
  line L11183 (-50.5065, -49.8409) -> (-50.5105, -49.9665)
  line L11184 (-39.6987, -52.2535) -> (-39.678, -52.0693)
  line L11185 (-39.6832, -52.4383) -> (-39.6987, -52.2535)
  line L11186 (-51.0703, -51.2327) -> (-51.2807, -51.4212)
  line L11187 (-51.5156, -51.5782) -> (-51.7703, -51.7005)
  line L11188 (-50.6837, -49.0179) -> (-50.5859, -49.2829)
  line L11189 (-38.0936, -52.9547) -> (-38.2397, -53.0689)
  line L11190 (-52.8813, -51.8055) -> (-53.1544, -51.7331)
  line L11191 (-54.3026, -48.961) -> (-54.1607, -48.7167)
  line L11192 (-53.0343, -47.9118) -> (-52.7572, -47.8567)
  line L11193 (-54.4086, -49.2229) -> (-54.3026, -48.961)
  line L11194 (-37.7991, -52.2933) -> (-37.8224, -52.4773)
  line L11195 (-39.1046, -51.386) -> (-38.9268, -51.3336)
  line L11196 (-39.4134, -51.588) -> (-39.2689, -51.4719)
  line L11197 (103.041, -53.7546) -> (102.879, -53.6642)
  line L11198 (-37.9725, -52.8144) -> (-38.0936, -52.9547)
  line L11199 (-51.9184, -47.9293) -> (-51.655, -48.0313)
  line L11200 (-50.8885, -51.0165) -> (-51.0703, -51.2327)
  line L11201 (-39.1291, -53.1373) -> (-39.2909, -53.0469)
  line L11202 (-39.5326, -51.7301) -> (-39.4134, -51.588)
  line L11203 (-38.5577, -51.3362) -> (-38.3806, -51.391)
  line L11204 (103.065, -52.0032) -> (103.243, -51.9509)
  line L11205 (102.756, -52.2053) -> (102.901, -52.0891)
  line L11206 (-38.9268, -51.3336) -> (-38.7421, -51.3168)
  line L11207 (-50.5481, -50.2465) -> (-50.6248, -50.5184)
  line L11208 (-46.9725, -49.9355) -> (-46.8296, -50.0536)
  line L11209 (102.738, -53.544) -> (102.622, -53.3987)
  line L11210 (-37.8224, -52.4773) -> (-37.8809, -52.6532)
  line L11211 (-39.4321, -52.9267) -> (-39.5473, -52.7814)
  line L11212 (-39.6219, -51.8925) -> (-39.5326, -51.7301)
  line L11213 (-51.4085, -48.1693) -> (-51.1839, -48.3407)
  line L11214 (-50.5859, -49.2829) -> (-50.5265, -49.5591)
  line L11215 (-39.678, -52.0693) -> (-39.6219, -51.8925)
  line L11216 (-54.3543, -50.6063) -> (-54.4437, -50.3383)
  line L11217 (-53.6565, -51.4772) -> (-53.8756, -51.2989)
  line L11218 (-50.739, -50.7768) -> (-50.8885, -51.0165)
  line L11219 (-54.0674, -51.0914) -> (-54.228, -50.859)
  line L11220 (-50.5265, -49.5591) -> (-50.5065, -49.8409)
  line L11221 (-52.3183, -51.832) -> (-52.6007, -51.8387)
  line L11222 (102.487, -53.0556) -> (102.471, -52.8708)
  line L11223 (103.243, -51.9509) -> (103.428, -51.9341)
  line L11224 (-39.2689, -51.4719) -> (-39.1046, -51.386)
  line L11225 (-38.9528, -53.1946) -> (-39.1291, -53.1373)
  line L11226 (-37.8169, -52.0823) -> (-37.7988, -52.2668)
  line L11227 (-50.9857, -48.542) -> (-50.8179, -48.7693)
  line L11228 (-53.1544, -51.7331) -> (-53.4145, -51.6229)
  line L11229 (-46.5718, -50.5385) -> (-46.5537, -50.723)
  line L11230 (-48.1871, -51.383) -> (-48.3022, -51.2377)
  line L11231 (-47.1602, -51.6088) -> (-47.3387, -51.6586)
  line L11232 (-46.5773, -50.9335) -> (-46.6358, -51.1094)
  line L11233 (-47.884, -51.5936) -> (-48.0459, -51.5031)
  line L11234 (-48.3769, -50.3488) -> (-48.2876, -50.1863)
  line L11235 (244.607, -46.2716) -> (244.882, -46.3354)
  line L11236 (-47.6817, -49.7899) -> (-47.4971, -49.7731)
  line L11237 (-53.4145, -51.6229) -> (-53.6565, -51.4772)
  line L11238 (-48.2876, -50.1863) -> (-48.1684, -50.0443)
  line L11239 (-48.3022, -51.2377) -> (-48.387, -51.0728)
  line L11240 (-48.4536, -50.7098) -> (-48.4329, -50.5255)
  line L11241 (245.617, -46.7468) -> (245.815, -46.9481)
  line L11242 (245.031, -50.1065) -> (244.761, -50.1917)
  line L11243 (245.731, -49.6388) -> (245.52, -49.8273)
  line L11244 (-51.7703, -51.7005) -> (-52.0396, -51.7857)
  line L11245 (-53.7814, -48.2999) -> (-53.5515, -48.1356)
  line L11246 (242.925, -49.7049) -> (242.733, -49.4975)
  line L11247 (245.52, -49.8273) -> (245.285, -49.9843)
  line L11248 (-47.1356, -49.8473) -> (-46.9725, -49.9355)
  line L11249 (-53.8756, -51.2989) -> (-54.0674, -51.0914)
  line L11250 (-46.8296, -50.0536) -> (-46.7124, -50.1973)
  line L11251 (244.2, -50.2448) -> (243.92, -50.2116)
  line L11252 (242.573, -49.2651) -> (242.447, -49.0124)
  line L11253 (-51.2807, -51.4212) -> (-51.5156, -51.5782)
  line L11254 (246.29, -48.3726) -> (246.253, -48.6526)
  line L11255 (246.294, -48.247) -> (246.29, -48.3726)
  line L11256 (-54.4767, -49.4971) -> (-54.4086, -49.2229)
  line L11257 (-54.4944, -50.0604) -> (-54.5055, -49.7781)
  line L11258 (-48.4381, -50.8945) -> (-48.4536, -50.7098)
  line L11259 (-47.5236, -51.6728) -> (-47.7077, -51.6509)
  line L11260 (244.761, -50.1917) -> (244.483, -50.2381)
  line L11261 (-48.4329, -50.5255) -> (-48.3769, -50.3488)
  line L11262 (245.392, -46.5754) -> (245.617, -46.7468)
  line L11263 (243.144, -49.8833) -> (242.925, -49.7049)
  line L11264 (246.253, -48.6526) -> (246.176, -48.9245)
  line L11265 (-52.6007, -51.8387) -> (-52.8813, -51.8055)
  line L11266 (-46.6358, -51.1094) -> (-46.7274, -51.2707)
  line L11267 (-47.8596, -49.8422) -> (-47.6817, -49.7899)
  line L11268 (-46.7274, -51.2707) -> (-46.8486, -51.411)
  line L11269 (-46.8486, -51.411) -> (-46.9947, -51.5252)
  line L11270 (-48.387, -51.0728) -> (-48.4381, -50.8945)
  line L11271 (-46.7124, -50.1973) -> (-46.6254, -50.361)
  line L11272 (243.647, -50.1392) -> (243.386, -50.029)
  line L11273 (-54.1607, -48.7167) -> (-53.9858, -48.4949)
  line L11274 (-52.7572, -47.8567) -> (-52.4751, -47.8412)
  line L11275 (-54.4437, -50.3383) -> (-54.4944, -50.0604)
  line L11276 (-48.0459, -51.5031) -> (-48.1871, -51.383)
  line L11277 (-48.0239, -49.9281) -> (-47.8596, -49.8422)
  line L11278 (-47.4971, -49.7731) -> (-47.3127, -49.7925)
  line L11279 (-47.7077, -51.6509) -> (-47.884, -51.5936)
  line L11280 (-48.1684, -50.0443) -> (-48.0239, -49.9281)
  line L11281 (-52.4751, -47.8412) -> (-52.1937, -47.8655)
  line L11282 (-47.3387, -51.6586) -> (-47.5236, -51.6728)
  line L11283 (-46.9947, -51.5252) -> (-47.1602, -51.6088)
  line L11284 (245.983, -47.1753) -> (246.117, -47.424)
  line L11285 (243.92, -50.2116) -> (243.647, -50.1392)
  line L11286 (-54.5055, -49.7781) -> (-54.4767, -49.4971)
  line L11287 (-46.5537, -50.723) -> (-46.5541, -50.7496)
  line L11288 (-46.6254, -50.361) -> (-46.5718, -50.5385)
  line L11289 (-46.5541, -50.7496) -> (-46.5773, -50.9335)
  line L11290 (244.882, -46.3354) -> (245.146, -46.4373)
  line L11291 (-47.3127, -49.7925) -> (-47.1356, -49.8473)
  line L11292 (244.326, -46.2472) -> (244.607, -46.2716)
  line L11293 (92.0186, -48.6125) -> (91.9419, -48.8844)
  line L11294 (245.146, -46.4373) -> (245.392, -46.5754)
  line L11295 (245.912, -49.4226) -> (245.731, -49.6388)
  line L11296 (242.295, -48.1842) -> (242.324, -47.9031)
  line L11297 (242.733, -49.4975) -> (242.573, -49.2651)
  line L11298 (243.386, -50.029) -> (243.144, -49.8833)
  line L11299 (242.447, -49.0124) -> (242.357, -48.7444)
  line L11300 (245.815, -46.9481) -> (245.983, -47.1753)
  line L11301 (90.373, -46.2316) -> (90.6482, -46.2953)
  line L11302 (91.6782, -49.3825) -> (91.4964, -49.5988)
  line L11303 (243.5, -46.4115) -> (243.767, -46.3179)
  line L11304 (91.3828, -46.7067) -> (91.581, -46.908)
  line L11305 (91.8277, -49.1428) -> (91.6782, -49.3825)
  line L11306 (89.0152, -46.5017) -> (89.2659, -46.3714)
  line L11307 (88.158, -47.5889) -> (88.2641, -47.3271)
  line L11308 (88.2124, -48.9723) -> (88.123, -48.7043)
  line L11309 (246.117, -47.424) -> (246.215, -47.689)
  line L11310 (91.4964, -49.5988) -> (91.286, -49.7872)
  line L11311 (89.2659, -46.3714) -> (89.5324, -46.2778)
  line L11312 (90.0916, -46.2072) -> (90.373, -46.2316)
  line L11313 (246.062, -49.1829) -> (245.912, -49.4226)
  line L11314 (90.2484, -50.1981) -> (89.9659, -50.2047)
  line L11315 (90.6482, -46.2953) -> (90.9117, -46.3973)
  line L11316 (89.8095, -46.2227) -> (90.0916, -46.2072)
  line L11317 (243.249, -46.5417) -> (243.5, -46.4115)
  line L11318 (239.966, -48.4597) -> (240.083, -48.6034)
  line L11319 (240.083, -48.6034) -> (240.17, -48.7671)
  line L11320 (91.7488, -47.1353) -> (91.883, -47.3839)
  line L11321 (92.0562, -48.3325) -> (92.0186, -48.6125)
  line L11322 (242.498, -47.3671) -> (242.64, -47.1228)
  line L11323 (239.483, -48.1985) -> (239.66, -48.2534)
  line L11324 (242.306, -48.4665) -> (242.295, -48.1842)
  line L11325 (88.4993, -49.4574) -> (88.3387, -49.225)
  line L11326 (88.7853, -46.6659) -> (89.0152, -46.5017)
  line L11327 (88.0722, -48.4264) -> (88.0611, -48.1441)
  line L11328 (91.581, -46.908) -> (91.7488, -47.1353)
  line L11329 (242.815, -46.901) -> (243.02, -46.706)
  line L11330 (243.767, -46.3179) -> (244.044, -46.2628)
  line L11331 (90.9117, -46.3973) -> (91.1582, -46.5353)
  line L11332 (91.9807, -47.6489) -> (92.0402, -47.9251)
  line L11333 (243.02, -46.706) -> (243.249, -46.5417)
  line L11334 (91.0511, -49.9442) -> (90.7964, -50.0665)
  line L11335 (242.324, -47.9031) -> (242.392, -47.629)
  line L11336 (88.0611, -48.1441) -> (88.0899, -47.8631)
  line L11337 (245.285, -49.9843) -> (245.031, -50.1065)
  line L11338 (91.9419, -48.8844) -> (91.8277, -49.1428)
  line L11339 (244.483, -50.2381) -> (244.2, -50.2448)
  line L11340 (242.357, -48.7444) -> (242.306, -48.4665)
  line L11341 (244.044, -46.2628) -> (244.326, -46.2472)
  line L11342 (92.0402, -47.9251) -> (92.0602, -48.2069)
  line L11343 (91.1582, -46.5353) -> (91.3828, -46.7067)
  line L11344 (90.7964, -50.0665) -> (90.527, -50.1517)
  line L11345 (239.66, -48.2534) -> (239.823, -48.3415)
  line L11346 (246.176, -48.9245) -> (246.062, -49.1829)
  line L11347 (89.5324, -46.2778) -> (89.8095, -46.2227)
  line L11348 (246.215, -47.689) -> (246.274, -47.9652)
  line L11349 (90.527, -50.1517) -> (90.2484, -50.1981)
  line L11350 (91.883, -47.3839) -> (91.9807, -47.6489)
  line L11351 (246.274, -47.9652) -> (246.294, -48.247)
  line L11352 (92.0602, -48.2069) -> (92.0562, -48.3325)
  line L11353 (242.392, -47.629) -> (242.498, -47.3671)
  line L11354 (242.64, -47.1228) -> (242.815, -46.901)
  line L11355 (91.286, -49.7872) -> (91.0511, -49.9442)
  line L11356 (238.911, -49.9997) -> (238.749, -49.9092)
  line L11357 (239.456, -50.0647) -> (239.272, -50.0789)
  line L11358 (238.608, -49.7891) -> (238.493, -49.6438)
  line L11359 (88.123, -48.7043) -> (88.0722, -48.4264)
  line L11360 (88.2641, -47.3271) -> (88.406, -47.0828)
  line L11361 (239.947, -49.8171) -> (239.801, -49.9312)
  line L11362 (88.9101, -49.8432) -> (88.6911, -49.6649)
  line L11363 (89.1522, -49.9889) -> (88.9101, -49.8432)
  line L11364 (95.8543, -48.5633) -> (95.9413, -48.727)
  line L11365 (239.801, -49.9312) -> (239.635, -50.0148)
  line L11366 (238.627, -48.4504) -> (238.771, -48.3342)
  line L11367 (238.749, -49.9092) -> (238.608, -49.7891)
  line L11368 (240.241, -49.1557) -> (240.218, -49.3396)
  line L11369 (238.508, -48.5924) -> (238.627, -48.4504)
  line L11370 (238.357, -49.3006) -> (238.342, -49.1159)
  line L11371 (240.159, -49.5155) -> (240.068, -49.6767)
  line L11372 (96.013, -49.0891) -> (96.0126, -49.1156)
  line L11373 (239.635, -50.0148) -> (239.456, -50.0647)
  line L11374 (238.342, -49.1159) -> (238.362, -48.9316)
  line L11375 (95.254, -48.1585) -> (95.4311, -48.2133)
  line L11376 (96.0126, -49.1156) -> (95.9894, -49.2995)
  line L11377 (238.418, -48.7549) -> (238.508, -48.5924)
  line L11378 (95.2279, -50.0246) -> (95.0431, -50.0389)
  line L11379 (94.1797, -49.4388) -> (94.1286, -49.2606)
  line L11380 (95.7371, -48.4197) -> (95.8543, -48.5633)
  line L11381 (238.362, -48.9316) -> (238.418, -48.7549)
  line L11382 (94.3796, -49.749) -> (94.2644, -49.6037)
  line L11383 (95.7181, -49.777) -> (95.572, -49.8912)
  line L11384 (95.0696, -48.1391) -> (95.254, -48.1585)
  line L11385 (94.7071, -48.2082) -> (94.885, -48.1559)
  line L11386 (88.0899, -47.8631) -> (88.158, -47.5889)
  line L11387 (240.218, -49.3396) -> (240.159, -49.5155)
  line L11388 (238.493, -49.6438) -> (238.408, -49.4788)
  line L11389 (239.823, -48.3415) -> (239.966, -48.4597)
  line L11390 (238.408, -49.4788) -> (238.357, -49.3006)
  line L11391 (95.4311, -48.2133) -> (95.5942, -48.3015)
  line L11392 (239.088, -50.057) -> (238.911, -49.9997)
  line L11393 (239.272, -50.0789) -> (239.088, -50.057)
  line L11394 (94.2644, -49.6037) -> (94.1797, -49.4388)
  line L11395 (89.4123, -50.0991) -> (89.1522, -49.9889)
  line L11396 (88.5809, -46.8609) -> (88.7853, -46.6659)
  line L11397 (89.9659, -50.2047) -> (89.6854, -50.1715)
  line L11398 (239.114, -48.196) -> (239.298, -48.1792)
  line L11399 (95.5942, -48.3015) -> (95.7371, -48.4197)
  line L11400 (95.8393, -49.6367) -> (95.7181, -49.777)
  line L11401 (238.936, -48.2483) -> (239.114, -48.196)
  line L11402 (240.242, -49.1291) -> (240.241, -49.1557)
  line L11403 (95.9949, -48.9045) -> (96.013, -49.0891)
  line L11404 (240.068, -49.6767) -> (239.947, -49.8171)
  line L11405 (94.5208, -49.8692) -> (94.3796, -49.749)
  line L11406 (95.572, -49.8912) -> (95.4065, -49.9748)
  line L11407 (94.6826, -49.9596) -> (94.5208, -49.8692)
  line L11408 (94.1898, -48.7148) -> (94.2791, -48.5523)
  line L11409 (88.406, -47.0828) -> (88.5809, -46.8609)
  line L11410 (95.9413, -48.727) -> (95.9949, -48.9045)
  line L11411 (95.9308, -49.4755) -> (95.8393, -49.6367)
  line L11412 (238.771, -48.3342) -> (238.936, -48.2483)
  line L11413 (94.885, -48.1559) -> (95.0696, -48.1391)
  line L11414 (88.3387, -49.225) -> (88.2124, -48.9723)
  line L11415 (239.298, -48.1792) -> (239.483, -48.1985)
  line L11416 (240.17, -48.7671) -> (240.223, -48.9446)
  line L11417 (88.6911, -49.6649) -> (88.4993, -49.4574)
  line L11418 (240.223, -48.9446) -> (240.242, -49.1291)
  line L11419 (89.6854, -50.1715) -> (89.4123, -50.0991)
  line L11420 (-56.5597, -48.9853) -> (-56.583, -49.1693)
  line L11421 (264.303, -45.3806) -> (264.55, -45.5187)
  line L11422 (-56.5774, -48.7743) -> (-56.5593, -48.9588)
  line L11423 (-58.3926, -49.3085) -> (-58.4437, -49.1303)
  line L11424 (94.5428, -48.2941) -> (94.7071, -48.2082)
  line L11425 (95.4065, -49.9748) -> (95.2279, -50.0246)
  line L11426 (263.919, -49.135) -> (263.64, -49.1814)
  line L11427 (94.1131, -49.0758) -> (94.1337, -48.8915)
  line L11428 (262.804, -49.0824) -> (262.544, -48.9723)
  line L11429 (-56.7181, -48.4331) -> (-56.631, -48.5968)
  line L11430 (-57.0003, -49.7609) -> (-57.1658, -49.8445)
  line L11431 (263.358, -49.188) -> (263.077, -49.1548)
  line L11432 (261.891, -48.4408) -> (261.73, -48.2084)
  line L11433 (261.73, -48.2084) -> (261.604, -47.9556)
  line L11434 (265.448, -47.3159) -> (265.41, -47.5958)
  line L11435 (261.604, -47.9556) -> (261.515, -47.6876)
  line L11436 (-57.8652, -48.078) -> (-57.6874, -48.0256)
  line L11437 (-58.4386, -48.7613) -> (-58.3825, -48.5845)
  line L11438 (264.973, -45.8914) -> (265.141, -46.1186)
  line L11439 (265.41, -47.5958) -> (265.334, -47.8677)
  line L11440 (-56.7331, -49.5064) -> (-56.8542, -49.6467)
  line L11441 (-58.3825, -48.5845) -> (-58.2932, -48.4221)
  line L11442 (-58.1927, -49.6187) -> (-58.3079, -49.4734)
  line L11443 (-56.6415, -49.3452) -> (-56.7331, -49.5064)
  line L11444 (-56.8542, -49.6467) -> (-57.0003, -49.7609)
  line L11445 (-58.2932, -48.4221) -> (-58.174, -48.28)
  line L11446 (-57.3444, -49.8943) -> (-57.5292, -49.9086)
  line L11447 (-58.3079, -49.4734) -> (-58.3926, -49.3085)
  line L11448 (94.1337, -48.8915) -> (94.1898, -48.7148)
  line L11449 (94.1286, -49.2606) -> (94.1131, -49.0758)
  line L11450 (-58.0515, -49.7389) -> (-58.1927, -49.6187)
  line L11451 (263.077, -49.1548) -> (262.804, -49.0824)
  line L11452 (265.219, -48.1261) -> (265.07, -48.3658)
  line L11453 (264.443, -48.9275) -> (264.188, -49.0498)
  line L11454 (261.464, -47.4097) -> (261.453, -47.1274)
  line L11455 (262.083, -48.6482) -> (261.891, -48.4408)
  line L11456 (263.64, -49.1814) -> (263.358, -49.188)
  line L11457 (-56.583, -49.1693) -> (-56.6415, -49.3452)
  line L11458 (95.0431, -50.0389) -> (94.859, -50.0169)
  line L11459 (94.859, -50.0169) -> (94.6826, -49.9596)
  line L11460 (-57.1412, -48.083) -> (-56.9781, -48.1712)
  line L11461 (-57.5027, -48.0088) -> (-57.3183, -48.0282)
  line L11462 (264.55, -45.5187) -> (264.775, -45.69)
  line L11463 (-58.174, -48.28) -> (-58.0295, -48.1639)